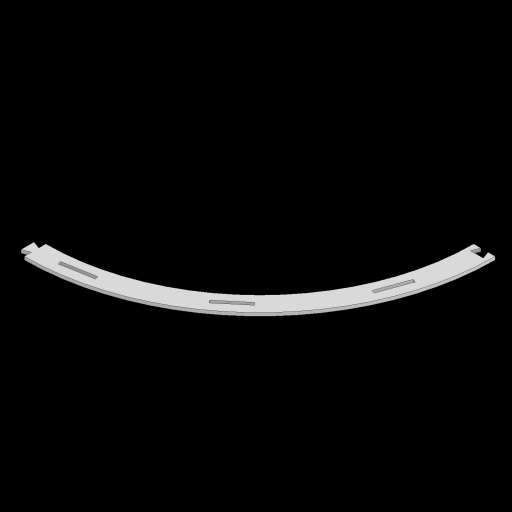
# Autodesk Inventor part: R0.2M
Saved by Autodesk Inventor 2024.2 (Build 282272000, 272)
## iProperties
Created: 2024-10-01
Part Number: R0.2M
Material: Generic
Document SubType Name: Modeling
Designer: jrcer
Density: 1 g/cm^3
Appearance: Default
Author: jrcer
Autodesk Inventor part; units mm, degrees
ref_plane "YZ Plane" through (0, 0, 0) normal (1, 0, 0) x (0, 1, 0)
ref_plane "XZ Plane" through (0, 0, 0) normal (0, 1, 0) x (-1, 0, 0)
ref_plane "XY Plane" through (0, 0, 0) normal (0, 0, 1) x (1, 0, 0)
sketch "Sketch1" plane through (0, 0, 0) normal (0, 1, 0) x (-1, 0, 0)
  circle A0 centre (0, 0) radius 200
  circle A1 centre (0, 0) radius 220
  line L0 (220, 0) -> (200, 0)
  line L1 (-220, 0) -> (-200, 0)
  line L2 (0, 0) -> (-200, 0) construction
  line L3 (0, 200) -> (0, 0) construction
  line L4 (0, 220) -> (0, 200)
  line L5 (-200, 0) -> (-220, 0)
  line L6 (-204, 7) -> (-216, 7)
  line L7 (-216, 7) -> (-213.4522, 0)
  line L8 (-204, 7) -> (-206.5478, 0)
  line L9 (-210, 0) -> (-210, 7) construction
  line L10 (-203.4647, 58.0945) -> (-193.2038, 86.2852)
  line L11 (-193.2038, 86.2852) -> (-190.1968, 85.1907)
  line L12 (-190.1968, 85.1907) -> (-200.4577, 57)
  line L13 (-200.4577, 57) -> (-203.4647, 58.0945)
  line L14 (-203.4647, 58.0945) -> (-190.1968, 85.1907) construction
  line L15 (-193.2038, 86.2852) -> (-200.4577, 57) construction
  circle A2 centre (0, 0) radius 210 construction
  line L16 (-7, -204) -> (0, -206.5478)
  line L17 (-7, -216) -> (0, -213.4522)
  line L18 (-7, -204) -> (-7, -216)
  line L19 (204, -7) -> (206.5478, 0)
  line L20 (216, -7) -> (213.4522, 0)
  line L21 (204, -7) -> (216, -7)
  line L22 (7, 204) -> (0, 206.5478)
  line L23 (7, 216) -> (0, 213.4522)
  line L24 (7, 204) -> (7, 216)
  line L25 (-205.2528, -51.421) -> (-210.462, -21.8768)
  line L26 (-202.1014, -50.8654) -> (-205.2528, -51.421)
  line L27 (-207.3106, -21.3211) -> (-202.1014, -50.8654)
  line L28 (-210.462, -21.8768) -> (-207.3106, -21.3211)
  line L29 (-152.0436, -147.1583) -> (-171.3271, -124.1768)
  line L30 (-149.5923, -145.1014) -> (-152.0436, -147.1583)
  line L31 (-168.8757, -122.1199) -> (-149.5923, -145.1014)
  line L32 (-171.3271, -124.1768) -> (-168.8757, -122.1199)
  line L33 (-58.0945, -203.4647) -> (-86.2852, -193.2038)
  line L34 (-57, -200.4577) -> (-58.0945, -203.4647)
  line L35 (-85.1907, -190.1968) -> (-57, -200.4577)
  line L36 (-86.2852, -193.2038) -> (-85.1907, -190.1968)
  line L37 (51.421, -205.2528) -> (21.8768, -210.462)
  line L38 (50.8654, -202.1014) -> (51.421, -205.2528)
  line L39 (21.3211, -207.3106) -> (50.8654, -202.1014)
  line L40 (21.8768, -210.462) -> (21.3211, -207.3106)
  line L41 (147.1583, -152.0436) -> (124.1768, -171.3271)
  line L42 (145.1014, -149.5923) -> (147.1583, -152.0436)
  line L43 (122.1199, -168.8757) -> (145.1014, -149.5923)
  line L44 (124.1768, -171.3271) -> (122.1199, -168.8757)
  line L45 (203.4647, -58.0945) -> (193.2038, -86.2852)
  line L46 (200.4577, -57) -> (203.4647, -58.0945)
  line L47 (190.1968, -85.1907) -> (200.4577, -57)
  line L48 (193.2038, -86.2852) -> (190.1968, -85.1907)
  line L49 (205.2528, 51.421) -> (210.462, 21.8768)
  line L50 (202.1014, 50.8654) -> (205.2528, 51.421)
  line L51 (207.3106, 21.3211) -> (202.1014, 50.8654)
  line L52 (210.462, 21.8768) -> (207.3106, 21.3211)
  line L53 (152.0436, 147.1583) -> (171.3271, 124.1768)
  line L54 (149.5923, 145.1014) -> (152.0436, 147.1583)
  line L55 (168.8757, 122.1199) -> (149.5923, 145.1014)
  line L56 (171.3271, 124.1768) -> (168.8757, 122.1199)
  line L57 (58.0945, 203.4647) -> (86.2852, 193.2038)
  line L58 (57, 200.4577) -> (58.0945, 203.4647)
  line L59 (85.1907, 190.1968) -> (57, 200.4577)
  line L60 (86.2852, 193.2038) -> (85.1907, 190.1968)
  line L61 (-51.421, 205.2528) -> (-21.8768, 210.462)
  line L62 (-50.8654, 202.1014) -> (-51.421, 205.2528)
  line L63 (-21.3211, 207.3106) -> (-50.8654, 202.1014)
  line L64 (-21.8768, 210.462) -> (-21.3211, 207.3106)
  line L65 (-147.1583, 152.0436) -> (-124.1768, 171.3271)
  line L66 (-145.1014, 149.5923) -> (-147.1583, 152.0436)
  line L67 (-122.1199, 168.8757) -> (-145.1014, 149.5923)
  line L68 (-124.1768, 171.3271) -> (-122.1199, 168.8757)
  point P0 (210, 0)
  point P1 (-210, 0)
  point P2 (-196.8307, 71.6426)
  point P3 (-40.1486, 206.1264)
  point P4 (-201.9612, 57.5472)
  point P5 (-191.7003, 85.7379)
  point P6 (-7, -210)
  point P7 (210, -7)
  point P8 (7, 210)
  point P9 (-203.6771, -51.1432)
  point P10 (-208.8863, -21.5989)
  point P11 (-150.818, -146.1299)
  point P12 (-170.1014, -123.1484)
  point P13 (-57.5472, -201.9612)
  point P14 (-85.7379, -191.7003)
  point P15 (51.1432, -203.6771)
  point P16 (21.5989, -208.8863)
  point P17 (146.1299, -150.818)
  point P18 (123.1484, -170.1014)
  point P19 (201.9612, -57.5472)
  point P20 (191.7003, -85.7379)
  point P21 (203.6771, 51.1432)
  point P22 (208.8863, 21.5989)
  point P23 (150.818, 146.1299)
  point P24 (170.1014, 123.1484)
  point P25 (57.5472, 201.9612)
  point P26 (85.7379, 191.7003)
  point P27 (-51.1432, 203.6771)
  point P28 (-21.5989, 208.8863)
  point P29 (-146.1299, 150.818)
  point P30 (-123.1484, 170.1014)
  point P31 (-206.5478, 0)
  point P32 (0, 206.5478)
  point P33 (0, 213.4522)
  dimension "d0" = 400
  dimension "d1" = 440
  dimension "d4" = 90
  dimension "d5" = 7
  dimension "d6" = 70
  dimension "d8" = 12
  dimension "d13" = 3.2
  dimension "d14" = 30
  dimension "d15" = 50
  dimension "d20" = 420
  dimension "d23" = 360
  dimension "d27" = 360
  constraints: 138 end point, 11 point on circle, 8 midpoint, 3 centre point, 3 coincident, 3 parallel, 2 horizontal, 2 horizontal alignment, 2 perpendicular, 2 point on line, 2 vertical, 1 collinear, 1 equal length, 154 other
  measures "d0" diameter of A0
  measures "d1" diameter of A1
  measures "d4" angle of L2 L3
  measures "d5" distance between parallel lines of L6 L5
  measures "d6" angle of L7 L6
  measures "d8" distance of L6.start L6.end
  measures "d13" distance of L10.end L11.end
  measures "d14" distance of L11.end L12.end
  measures "d15" vertical distance of L12.end L6.start
  measures "d20" diameter of A2
extrude "Extrusion1" add sketch "Sketch1" along normal blind 3 contours A0 L1 L8 L6 L7 A1 L4 | L4 L23 L24 L22
body "Solid1"
